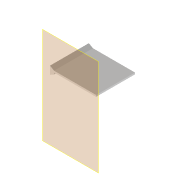
# Autodesk Inventor part: IM_ledmatrix_diffuser
Saved by Autodesk Inventor 2022 (Build 260153000, 153)
## iProperties
Created: 2023-06-20
Part Number: IM_ledmatrix_diffuser
Material: Generisch
Document SubType Name: Modeling
Designer: diederichbenedict
Density: 1 g/cm^3
Appearance: Vorgabe
Author: diederichbenedict
Autodesk Inventor part; units mm, degrees
ref_plane "YZ Plane" through (0, 0, 0) normal (1, 0, 0) x (0, 1, 0)
ref_plane "XZ Plane" through (0, 0, 0) normal (0, 1, 0) x (-1, 0, 0)
ref_plane "XY Plane" through (0, 0, 0) normal (0, 0, 1) x (1, 0, 0)
ref_plane "Arbeitsebene1" through (0, 0, 0) normal (0, 0, 1) x (1, 0, 0)
sketch "Skizze1" plane through (0, 0, 0) normal (0, 0, 1) x (1, 0, 0)
  line L0 (4.5, 37.1634) -> (3, 36.2973) projected
  line L1 (3, 36.2973) -> (3, 42.1841) projected
  line L2 (3, 42.1841) -> (4.5, 41.3181) projected
  line L3 (4.5, 41.3181) -> (4.5, 50) projected
  line L4 (3.1236, 50) -> (4.5, 50) projected
  line L5 (3.1236, 50) -> (3.1236, 53) projected
  line L6 (3.1236, 53) -> (33.1236, 53) projected
  line L7 (33.1236, 53) -> (33.1236, 57) projected
  line L8 (0, 57) -> (33.1236, 57) projected
  line L9 (0, 0) -> (0, 57) projected
  line L10 (0, 0) -> (4.5, 0) projected
  line L11 (4.5, 0) -> (4.5, 37.1634) projected
  line L12 (4.5, 37.1634) -> (5.5, 37.7407) projected
  line L13 (5.5, 37.7407) -> (6.5, 37.7407) projected
  line L14 (6.5, 40.7407) -> (5.5, 40.7407) projected
  line L15 (5.5, 40.7407) -> (4.5, 41.3181) projected
  line L16 (4.4, 41.1449) -> (3.2, 41.8377)
  line L17 (3.2, 41.8377) -> (3.2, 36.6437)
  line L18 (3.2, 36.6437) -> (4.4, 37.3366)
  line L19 (4.4, 41.1449) -> (6.8321, 39.7407)
  line L20 (6.8321, 39.7407) -> (6.8321, 38.7407)
  line L21 (6.8321, 38.7407) -> (4.4, 37.3366)
  line L22 (33.1236, 40.3183) -> (33.1236, 39.2407)
  line L23 (33.1236, 39.2407) -> (6.8321, 39.2407)
  line L24 (33.1236, 39.2407) -> (6.8321, 39.2407)
  line L25 (6.8321, 39.2407) -> (6.8321, 38.7407)
  line L26 (6.8321, 38.7407) -> (33.1236, 38.7407)
  line L27 (33.1236, 38.7407) -> (33.1236, 39.2407)
  line L28 (6.8321, 38.7407) -> (3.2, 38.7407)
  dimension "d0" = 0.2
  dimension "d3" = 0.5
  dimension "d4" = 1.4042
  constraints: 26 end point, 2 parallel, 2 perpendicular, 2 point on line, 1 horizontal, 1 midpoint, 1 vertical, 3 other
  measures "d0" distance between parallel lines of L2 L16
  measures "d3" distance between parallel lines of L26 L23
  measures "d4" vertical distance of L20.end L21.end
ref_plane "Arbeitsebene2" through (-0.0423, 0, -25.2444) normal (0, 0, -1) x (0, 1, 0)
extrude "Extrusion1" add sketch "Skizze1" against normal up to surface (25.2444 mm away) contours L19 L20 L28 L17 L16 | L23 L27 L26 L20
